SLMS LOGO (Autodesk Fusion 360 design; units mm, degrees)
Autodesk Fusion 360 part; units mm, degrees
sketch "Sketch1" plane through (0, 0, 0) normal (0, 1, 0) x (1, 0, 0)
  line L0 (0, 0) -> (135.4667, 0)
  line L1 (135.4667, 0) -> (135.4667, -135.4667)
  line L2 (135.4667, -135.4667) -> (0, -135.4667)
  line L3 (0, -135.4667) -> (0, 0)
  line L4 (27.5167, -27.5167) -> (48.6833, -27.5167)
  line L5 (48.6833, -27.5167) -> (65.8283, -56.0917)
  line L6 (65.8283, -56.0917) -> (53.1283, -77.2583)
  line L7 (53.1283, -77.2583) -> (48.6833, -69.85)
  line L8 (48.6833, -69.85) -> (48.6833, -107.95)
  line L9 (48.6833, -107.95) -> (27.5167, -107.95)
  line L10 (27.5167, -107.95) -> (27.5167, -103.7167)
  line L11 (27.5167, -103.7167) -> (31.75, -103.7167)
  line L12 (31.75, -103.7167) -> (31.75, -101.6)
  line L13 (31.75, -101.6) -> (27.5167, -101.6)
  line L14 (27.5167, -101.6) -> (27.5167, -97.3667)
  line L15 (27.5167, -97.3667) -> (35.9833, -97.3667)
  line L16 (35.9833, -97.3667) -> (35.9833, -95.25)
  line L17 (35.9833, -95.25) -> (27.5167, -95.25)
  line L18 (27.5167, -95.25) -> (27.5167, -91.0167)
  line L19 (27.5167, -91.0167) -> (31.75, -91.0167)
  line L20 (31.75, -91.0167) -> (31.75, -88.9)
  line L21 (31.75, -88.9) -> (27.5167, -88.9)
  line L22 (27.5167, -88.9) -> (27.5167, -84.6667)
  line L23 (27.5167, -84.6667) -> (31.75, -84.6667)
  line L24 (31.75, -84.6667) -> (31.75, -82.55)
  line L25 (31.75, -82.55) -> (27.5167, -82.55)
  line L26 (27.5167, -82.55) -> (27.5167, -78.3167)
  line L27 (27.5167, -78.3167) -> (35.9833, -78.3167)
  line L28 (35.9833, -78.3167) -> (35.9833, -76.2)
  line L29 (35.9833, -76.2) -> (27.5167, -76.2)
  line L30 (27.5167, -76.2) -> (27.5167, -71.9667)
  line L31 (27.5167, -71.9667) -> (31.75, -71.9667)
  line L32 (31.75, -71.9667) -> (31.75, -69.85)
  line L33 (31.75, -69.85) -> (27.5167, -69.85)
  line L34 (27.5167, -69.85) -> (27.5167, -65.6167)
  line L35 (27.5167, -65.6167) -> (31.75, -65.6167)
  line L36 (31.75, -65.6167) -> (31.75, -63.5)
  line L37 (31.75, -63.5) -> (27.5167, -63.5)
  line L38 (27.5167, -63.5) -> (27.5167, -59.2667)
  line L39 (27.5167, -59.2667) -> (35.9833, -59.2667)
  line L40 (35.9833, -59.2667) -> (35.9833, -57.15)
  line L41 (35.9833, -57.15) -> (27.5167, -57.15)
  line L42 (27.5167, -57.15) -> (27.5167, -52.9167)
  line L43 (27.5167, -52.9167) -> (31.75, -52.9167)
  line L44 (31.75, -52.9167) -> (31.75, -50.8)
  line L45 (31.75, -50.8) -> (27.5167, -50.8)
  line L46 (27.5167, -50.8) -> (27.5167, -46.5667)
  line L47 (27.5167, -46.5667) -> (31.75, -46.5667)
  line L48 (31.75, -46.5667) -> (31.75, -44.45)
  line L49 (31.75, -44.45) -> (27.5167, -44.45)
  line L50 (27.5167, -44.45) -> (27.5167, -40.2167)
  line L51 (27.5167, -40.2167) -> (35.9833, -40.2167)
  line L52 (35.9833, -40.2167) -> (35.9833, -38.1)
  line L53 (35.9833, -38.1) -> (27.5167, -38.1)
  line L54 (27.5167, -38.1) -> (27.5167, -33.8667)
  line L55 (27.5167, -33.8667) -> (31.75, -33.8667)
  line L56 (31.75, -33.8667) -> (31.75, -31.75)
  line L57 (31.75, -31.75) -> (27.5167, -31.75)
  line L58 (27.5167, -31.75) -> (27.5167, -27.5167)
  line L59 (86.7833, -27.5167) -> (55.0333, -80.4333)
  line L60 (55.0333, -80.4333) -> (67.7333, -101.6)
  line L61 (67.7333, -101.6) -> (86.7833, -69.85)
  line L62 (86.7833, -69.85) -> (86.7833, -107.95)
  line L63 (86.7833, -107.95) -> (107.95, -107.95)
  line L64 (107.95, -107.95) -> (107.95, -27.5167)
  line L65 (107.95, -27.5167) -> (86.7833, -27.5167)
  spline S0 degree 3 poles (67.7333, -82.55) (66.5692, -82.55) (65.6167, -81.5975) (65.6167, -80.4333) knots 0 0 0 0 1 1 1 1
  spline S1 degree 3 poles (65.6167, -80.4333) (65.6167, -79.2692) (66.5692, -78.3167) (67.7333, -78.3167) knots 0 0 0 0 1 1 1 1
  spline S2 degree 3 poles (67.7333, -78.3167) (68.8975, -78.3167) (69.85, -79.2692) (69.85, -80.4333) knots 0 0 0 0 1 1 1 1
  spline S3 degree 3 poles (69.85, -80.4333) (69.85, -81.5975) (68.8975, -82.55) (67.7333, -82.55) knots 0 0 0 0 1 1 1 1
  spline S4 degree 3 poles (99.4833, -97.3667) (99.4833, -98.5308) (98.5308, -99.4833) (97.3667, -99.4833) knots 0 0 0 0 1 1 1 1
  spline S5 degree 3 poles (97.3667, -99.4833) (96.2025, -99.4833) (95.25, -98.5308) (95.25, -97.3667) knots 0 0 0 0 1 1 1 1
  line L66 (95.25, -97.3667) -> (95.25, -38.1)
  spline S6 degree 3 poles (95.25, -38.1) (95.25, -36.9358) (96.2025, -35.9833) (97.3667, -35.9833) knots 0 0 0 0 1 1 1 1
  spline S7 degree 3 poles (97.3667, -35.9833) (98.5308, -35.9833) (99.4833, -36.9358) (99.4833, -38.1) knots 0 0 0 0 1 1 1 1
  line L67 (99.4833, -38.1) -> (99.4833, -97.3667)
extrude "Extrude1" add sketch "Sketch1" along normal blind 1 contours L4 L5 L6 L7 L8 L9 L10 L11 L12 L13 L14 L15 L16 L17 L18 L19 L20 L21 L22 L23 L24 L25 L26 L27 L28 L29 L30 L31 L32 L33 L34 L35 L36 L37 L38 L39 L40 L41 L42 L43 L44 L45 L46 L47 L48 L49 L50 L51 L52 L53 L54 L55 L56 L57 L58 | L59 L60 L61 L62 L63 L64 L65 makes body 1 at (50.165, 0, 41.275) makes body 2 at (80.3595, 0, 58.565)
scale "Scale1" factor 2.5 about (55.0333, 1, 80.4333) bodies 1 2
scale "Scale2" factor 0.8 about (86.7833, -1.5, 75.1417) bodies 1 2
sketch "Sketch2" plane through (0, 0.5, 0) normal (0, 1, 0) x (-1, 0, 0)
sketch "Sketch3" plane through (0, 0.5, 0) normal (0, 1, 0) x (-1, 0, 0)
  circle A0 centre (-10.5, -22.5) radius 2.5
  circle A1 centre (-36, -22.5) radius 2.5
  circle A2 centre (-138, -22.5) radius 2.5
  circle A3 centre (-163.5, -22.5) radius 2.5
  circle A4 centre (-10.5, -9.75) radius 2.5
  circle A5 centre (-36, -9.75) radius 2.5
  circle A6 centre (-138, -9.75) radius 2.5
  circle A7 centre (-163.5, -9.75) radius 2.5
  circle A8 centre (-10.5, 3) radius 2.5
  circle A9 centre (-36, 3) radius 2.5
  circle A10 centre (-61.5, 3) radius 2.5
  circle A11 centre (-112.5, 3) radius 2.5
  circle A12 centre (-138, 3) radius 2.5
  circle A13 centre (-163.5, 3) radius 2.5
  circle A14 centre (-10.5, 15.75) radius 2.5
  circle A15 centre (-36, 15.75) radius 2.5
  circle A16 centre (-61.5, 15.75) radius 2.5
  circle A17 centre (-112.5, 15.75) radius 2.5
  circle A18 centre (-138, 15.75) radius 2.5
  circle A19 centre (-163.5, 15.75) radius 2.5
  circle A20 centre (-10.5, 28.5) radius 2.5
  circle A21 centre (-36, 28.5) radius 2.5
  circle A22 centre (-61.5, 28.5) radius 2.5
  circle A23 centre (-112.5, 28.5) radius 2.5
  circle A24 centre (-138, 28.5) radius 2.5
  circle A25 centre (-163.5, 28.5) radius 2.5
  circle A26 centre (-10.5, 41.25) radius 2.5
  circle A27 centre (-36, 41.25) radius 2.5
  circle A28 centre (-61.5, 41.25) radius 2.5
  circle A29 centre (-112.5, 41.25) radius 2.5
  circle A30 centre (-138, 41.25) radius 2.5
  circle A31 centre (-163.5, 41.25) radius 2.5
  circle A32 centre (-10.5, 54) radius 2.5
  circle A33 centre (-36, 54) radius 2.5
  circle A34 centre (-61.5, 54) radius 2.5
  circle A35 centre (-87, 54) radius 2.5
  circle A36 centre (-112.5, 54) radius 2.5
  circle A37 centre (-138, 54) radius 2.5
  circle A38 centre (-163.5, 54) radius 2.5
  circle A39 centre (-10.5, 66.75) radius 2.5
  circle A40 centre (-36, 66.75) radius 2.5
  circle A41 centre (-87, 66.75) radius 2.5
  circle A42 centre (-112.5, 66.75) radius 2.5
  circle A43 centre (-138, 66.75) radius 2.5
  circle A44 centre (-163.5, 66.75) radius 2.5
  circle A45 centre (-10.5, 79.5) radius 2.5
  circle A46 centre (-36, 79.5) radius 2.5
  circle A47 centre (-138, 79.5) radius 2.5
  circle A48 centre (-163.5, 79.5) radius 2.5
  circle A49 centre (-10.5, 92.25) radius 2.5
  circle A50 centre (-36, 92.25) radius 2.5
  circle A51 centre (-87, 92.25) radius 2.5
  circle A52 centre (-138, 92.25) radius 2.5
  circle A53 centre (-163.5, 92.25) radius 2.5
  circle A54 centre (-10.5, 105) radius 2.5
  circle A55 centre (-36, 105) radius 2.5
  circle A56 centre (-87, 105) radius 2.5
  circle A57 centre (-138, 105) radius 2.5
  circle A58 centre (-163.5, 105) radius 2.5
  circle A59 centre (-10.5, 117.75) radius 2.5
  circle A60 centre (-36, 117.75) radius 2.5
  circle A61 centre (-138, 117.75) radius 2.5
  circle A62 centre (-163.5, 117.75) radius 2.5
  circle A63 centre (-10.5, 130.5) radius 2.5
  circle A64 centre (-36, 130.5) radius 2.5
  circle A65 centre (-138, 130.5) radius 2.5
  circle A66 centre (-163.5, 130.5) radius 2.5
  dimension "d11" = 5
  dimension "d14" = -153
  dimension "d15" = 153
  measures "d11" diameter of A0
sketch "Sketch8" plane through (0, 0.5, 0) normal (0, 1, 0) x (-1, 0, 0)
  line L0 (-6.35, -17.9917) -> (-14.8167, -17.9917)
  line L1 (-14.8167, -17.9917) -> (-14.8167, -13.7583)
  line L2 (-14.8167, -13.7583) -> (-6.35, -13.7583)
  line L3 (-6.35, -13.7583) -> (-6.35, -5.2917)
  line L4 (-6.35, -5.2917) -> (-23.2833, -5.2917)
  line L5 (-23.2833, -5.2917) -> (-23.2833, -1.0583)
  line L6 (-23.2833, -1.0583) -> (-6.35, -1.0583)
  line L7 (-6.35, -1.0583) -> (-6.35, 7.4083)
  line L8 (-6.35, 7.4083) -> (-14.8167, 7.4083)
  line L9 (-14.8167, 7.4083) -> (-14.8167, 11.6417)
  line L10 (-14.8167, 11.6417) -> (-6.35, 11.6417)
  line L11 (-6.35, 11.6417) -> (-6.35, 20.1083)
  line L12 (-6.35, 20.1083) -> (-14.8167, 20.1083)
  line L13 (-14.8167, 20.1083) -> (-14.8167, 24.3417)
  line L14 (-14.8167, 24.3417) -> (-6.35, 24.3417)
  line L15 (-6.35, 24.3417) -> (-6.35, 32.8083)
  line L16 (-6.35, 32.8083) -> (-23.2833, 32.8083)
  line L17 (-23.2833, 32.8083) -> (-23.2833, 37.0417)
  line L18 (-23.2833, 37.0417) -> (-6.35, 37.0417)
  line L19 (-6.35, 37.0417) -> (-6.35, 45.5083)
  line L20 (-6.35, 45.5083) -> (-14.8167, 45.5083)
  line L21 (-14.8167, 45.5083) -> (-14.8167, 49.7417)
  line L22 (-14.8167, 49.7417) -> (-6.35, 49.7417)
  line L23 (-6.35, 49.7417) -> (-6.35, 58.2083)
  line L24 (-6.35, 58.2083) -> (-14.8167, 58.2083)
  line L25 (-14.8167, 58.2083) -> (-14.8167, 62.4417)
  line L26 (-14.8167, 62.4417) -> (-6.35, 62.4417)
  line L27 (-6.35, 62.4417) -> (-6.35, 70.9083)
  line L28 (-6.35, 70.9083) -> (-23.2833, 70.9083)
  line L29 (-23.2833, 70.9083) -> (-23.2833, 75.1417)
  line L30 (-23.2833, 75.1417) -> (-6.35, 75.1417)
  line L31 (-6.35, 75.1417) -> (-6.35, 83.6083)
  line L32 (-6.35, 83.6083) -> (-14.8167, 83.6083)
  line L33 (-14.8167, 83.6083) -> (-14.8167, 87.8417)
  line L34 (-14.8167, 87.8417) -> (-6.35, 87.8417)
  line L35 (-6.35, 87.8417) -> (-6.35, 96.3083)
  line L36 (-6.35, 96.3083) -> (-14.8167, 96.3083)
  line L37 (-14.8167, 96.3083) -> (-14.8167, 100.5417)
  line L38 (-14.8167, 100.5417) -> (-6.35, 100.5417)
  line L39 (-6.35, 100.5417) -> (-6.35, 109.0083)
  line L40 (-6.35, 109.0083) -> (-23.2833, 109.0083)
  line L41 (-23.2833, 109.0083) -> (-23.2833, 113.2417)
  line L42 (-23.2833, 113.2417) -> (-6.35, 113.2417)
  line L43 (-6.35, 113.2417) -> (-6.35, 121.7083)
  line L44 (-6.35, 121.7083) -> (-14.8167, 121.7083)
  line L45 (-14.8167, 121.7083) -> (-14.8167, 125.9417)
  line L46 (-14.8167, 125.9417) -> (-6.35, 125.9417)
  line L47 (-6.35, 125.9417) -> (-6.35, 134.4083)
  line L48 (-6.35, 134.4083) -> (-48.6833, 134.4083)
  line L49 (-48.6833, 134.4083) -> (-48.6833, 58.2083)
  line L50 (-48.6833, 58.2083) -> (-57.5733, 73.025)
  line L51 (-57.5733, 73.025) -> (-82.9733, 30.6917)
  line L52 (-82.9733, 30.6917) -> (-48.6833, -26.4583)
  line L53 (-48.6833, -26.4583) -> (-6.35, -26.4583)
  line L54 (-6.35, -26.4583) -> (-6.35, -17.9917)
  line L55 (-6.35, 134.4083) -> (-167.2167, 134.4083)
  line L56 (-167.2167, 134.4083) -> (-167.2167, 144.4083)
  line L57 (-167.2167, 144.4083) -> (-6.35, 144.4083)
  line L58 (-6.35, 144.4083) -> (-6.35, 134.4083)
  dimension "d39" = 10
  constraint horizontal L55
  constraint vertical L56
  constraint horizontal L57
  constraint vertical L58
  constraint coincident L47.end L48.start
  measures "d39" distance of L47.end L57.end
extrude "Extrude9" add sketch "Sketch8" against normal blind 40 separate body contours L48 L55 L56 L57 L58 makes body 3
sketch "Sketch4" plane through (0, 0.5, 0) normal (0, 1, 0) x (-1, 0, 0)
  circle A0 centre (-23, -10) radius 1.5
  circle A1 centre (-48.5, -10) radius 1.5
  circle A2 centre (-125, -10) radius 1.5
  circle A3 centre (-150.5, -10) radius 1.5
  circle A4 centre (-23, 15.5) radius 1.5
  circle A5 centre (-48.5, 15.5) radius 1.5
  circle A6 centre (-125, 15.5) radius 1.5
  circle A7 centre (-23, 41) radius 1.5
  circle A8 centre (-48.5, 41) radius 1.5
  circle A9 centre (-74, 41) radius 1.5
  circle A10 centre (-99.5, 41) radius 1.5
  circle A11 centre (-125, 41) radius 1.5
  circle A12 centre (-23, 66.5) radius 1.5
  circle A13 centre (-74, 66.5) radius 1.5
  circle A14 centre (-99.5, 66.5) radius 1.5
  circle A15 centre (-23, 92) radius 1.5
  circle A16 centre (-74, 92) radius 1.5
  circle A17 centre (-99.5, 92) radius 1.5
  circle A18 centre (-23, 117.5) radius 1.5
  circle A19 centre (-150.5, 117.5) radius 1.5
  point P0 (-10.5, -22.5)
  dimension "d17" = 3
  dimension "d20" = -153
  dimension "d21" = 153
  measures "d17" diameter of A0
extrude "Extrude4" [suppressed]
shell "Shell2" [suppressed]
extrude "Extrude5" [suppressed]
extrude "Extrude6" [suppressed]
sketch "Sketch7" plane through (0, -1.5, 0) normal (0, -1, 0) x (1, 0, 0)
  arc A0 (12.809, 118.7083) -> (12.4937, 116.2417) centre (10.5, 117.75) ccw
  line L0 (12.809, 118.7083) -> (17.8167, 118.7083)
  line L1 (17.8167, 118.7083) -> (17.8167, 128.9417)
  line L2 (17.8167, 128.9417) -> (12.4549, 128.9417)
  arc A1 (12.8291, 131.4083) -> (12.4549, 128.9417) centre (10.5, 130.5) ccw
  line L3 (12.8291, 131.4083) -> (33.6709, 131.4083)
  arc A2 (38.3291, 131.4083) -> (33.6709, 131.4083) centre (36, 130.5) ccw
  line L4 (38.3291, 131.4083) -> (45.6833, 131.4083)
  line L5 (45.6833, 131.4083) -> (45.6833, 47.3774)
  line L6 (45.6833, 47.3774) -> (57.5733, 67.194)
  line L7 (57.5733, 67.194) -> (72.7725, 41.8621)
  arc A3 (74.183, 39.5112) -> (72.7725, 41.8621) centre (74, 41) ccw
  line L8 (74.183, 39.5112) -> (79.4748, 30.6917)
  line L9 (79.4748, 30.6917) -> (63.6376, 4.2964)
  arc A4 (61.362, 0.5038) -> (63.6376, 4.2964) centre (61.5, 3) ccw
  line L10 (61.362, 0.5038) -> (46.9848, -23.4583)
  line L11 (46.9848, -23.4583) -> (38.309, -23.4583)
  arc A5 (33.691, -23.4583) -> (38.309, -23.4583) centre (36, -22.5) ccw
  line L12 (33.691, -23.4583) -> (12.809, -23.4583)
  arc A6 (12.4937, -20.9917) -> (12.809, -23.4583) centre (10.5, -22.5) ccw
  line L13 (12.4937, -20.9917) -> (17.8167, -20.9917)
  line L14 (17.8167, -20.9917) -> (17.8167, -10.7583)
  line L15 (17.8167, -10.7583) -> (12.7876, -10.7583)
  arc A7 (12.5306, -8.2917) -> (12.7876, -10.7583) centre (10.5, -9.75) ccw
  line L16 (12.5306, -8.2917) -> (26.2833, -8.2917)
  line L17 (26.2833, -8.2917) -> (26.2833, 1.9417)
  line L18 (26.2833, 1.9417) -> (12.7649, 1.9417)
  arc A8 (12.5656, 4.4083) -> (12.7649, 1.9417) centre (10.5, 3) ccw
  line L19 (12.5656, 4.4083) -> (17.8167, 4.4083)
  line L20 (17.8167, 4.4083) -> (17.8167, 14.6417)
  line L21 (17.8167, 14.6417) -> (12.7409, 14.6417)
  arc A9 (12.5988, 17.1083) -> (12.7409, 14.6417) centre (10.5, 15.75) ccw
  line L22 (12.5988, 17.1083) -> (17.8167, 17.1083)
  line L23 (17.8167, 17.1083) -> (17.8167, 27.3417)
  line L24 (17.8167, 27.3417) -> (12.7155, 27.3417)
  arc A10 (12.6303, 29.8083) -> (12.7155, 27.3417) centre (10.5, 28.5) ccw
  line L25 (12.6303, 29.8083) -> (26.2833, 29.8083)
  line L26 (26.2833, 29.8083) -> (26.2833, 40.0417)
  line L27 (26.2833, 40.0417) -> (24.1539, 40.0417)
  arc A11 (21.8461, 40.0417) -> (24.1539, 40.0417) centre (23, 41) ccw
  line L28 (21.8461, 40.0417) -> (12.6886, 40.0417)
  arc A12 (12.6602, 42.5083) -> (12.6886, 40.0417) centre (10.5, 41.25) ccw
  line L29 (12.6602, 42.5083) -> (17.8167, 42.5083)
  line L30 (17.8167, 42.5083) -> (17.8167, 52.7417)
  line L31 (17.8167, 52.7417) -> (12.6602, 52.7417)
  arc A13 (12.6886, 55.2083) -> (12.6602, 52.7417) centre (10.5, 54) ccw
  line L32 (12.6886, 55.2083) -> (17.8167, 55.2083)
  line L33 (17.8167, 55.2083) -> (17.8167, 65.4417)
  line L34 (17.8167, 65.4417) -> (12.6303, 65.4417)
  arc A14 (12.7155, 67.9083) -> (12.6303, 65.4417) centre (10.5, 66.75) ccw
  line L35 (12.7155, 67.9083) -> (22.4837, 67.9083)
  arc A15 (23.5163, 67.9083) -> (22.4837, 67.9083) centre (23, 66.5) ccw
  line L36 (23.5163, 67.9083) -> (26.2833, 67.9083)
  line L37 (26.2833, 67.9083) -> (26.2833, 78.1417)
  line L38 (26.2833, 78.1417) -> (12.5988, 78.1417)
  arc A16 (12.7409, 80.6083) -> (12.5988, 78.1417) centre (10.5, 79.5) ccw
  line L39 (12.7409, 80.6083) -> (17.8167, 80.6083)
  line L40 (17.8167, 80.6083) -> (17.8167, 90.8417)
  line L41 (17.8167, 90.8417) -> (12.5656, 90.8417)
  arc A17 (12.7649, 93.3083) -> (12.5656, 90.8417) centre (10.5, 92.25) ccw
  line L42 (12.7649, 93.3083) -> (17.8167, 93.3083)
  line L43 (17.8167, 93.3083) -> (17.8167, 103.5417)
  line L44 (17.8167, 103.5417) -> (12.5306, 103.5417)
  arc A18 (12.7876, 106.0083) -> (12.5306, 103.5417) centre (10.5, 105) ccw
  line L45 (12.7876, 106.0083) -> (26.2833, 106.0083)
  line L46 (26.2833, 106.0083) -> (26.2833, 116.2417)
  line L47 (26.2833, 116.2417) -> (23.8165, 116.2417)
  arc A19 (22.1835, 116.2417) -> (23.8165, 116.2417) centre (23, 117.5) ccw
  line L48 (22.1835, 116.2417) -> (12.4937, 116.2417)
  line L49 (14.8167, -17.9917) -> (6.35, -17.9917)
  line L50 (6.35, -17.9917) -> (6.35, -26.4583)
  line L51 (6.35, -26.4583) -> (48.6833, -26.4583)
  line L52 (48.6833, -26.4583) -> (82.9733, 30.6917)
  line L53 (82.9733, 30.6917) -> (57.5733, 73.025)
  line L54 (57.5733, 73.025) -> (48.6833, 58.2083)
  line L55 (48.6833, 58.2083) -> (48.6833, 134.4083)
  line L56 (48.6833, 134.4083) -> (6.35, 134.4083)
  line L57 (6.35, 134.4083) -> (6.35, 125.9417)
  line L58 (6.35, 125.9417) -> (14.8167, 125.9417)
  line L59 (14.8167, 125.9417) -> (14.8167, 121.7083)
  line L60 (14.8167, 121.7083) -> (6.35, 121.7083)
  line L61 (6.35, 121.7083) -> (6.35, 113.2417)
  line L62 (6.35, 113.2417) -> (23.2833, 113.2417)
  line L63 (23.2833, 113.2417) -> (23.2833, 109.0083)
  line L64 (23.2833, 109.0083) -> (6.35, 109.0083)
  line L65 (6.35, 109.0083) -> (6.35, 100.5417)
  line L66 (6.35, 100.5417) -> (14.8167, 100.5417)
  line L67 (14.8167, 100.5417) -> (14.8167, 96.3083)
  line L68 (14.8167, 96.3083) -> (6.35, 96.3083)
  line L69 (6.35, 96.3083) -> (6.35, 87.8417)
  line L70 (6.35, 87.8417) -> (14.8167, 87.8417)
  line L71 (14.8167, 87.8417) -> (14.8167, 83.6083)
  line L72 (14.8167, 83.6083) -> (6.35, 83.6083)
  line L73 (6.35, 83.6083) -> (6.35, 75.1417)
  line L74 (6.35, 75.1417) -> (23.2833, 75.1417)
  line L75 (23.2833, 75.1417) -> (23.2833, 70.9083)
  line L76 (23.2833, 70.9083) -> (6.35, 70.9083)
  line L77 (6.35, 70.9083) -> (6.35, 62.4417)
  line L78 (6.35, 62.4417) -> (14.8167, 62.4417)
  line L79 (14.8167, 62.4417) -> (14.8167, 58.2083)
  line L80 (14.8167, 58.2083) -> (6.35, 58.2083)
  line L81 (6.35, 58.2083) -> (6.35, 49.7417)
  line L82 (6.35, 49.7417) -> (14.8167, 49.7417)
  line L83 (14.8167, 49.7417) -> (14.8167, 45.5083)
  line L84 (14.8167, 45.5083) -> (6.35, 45.5083)
  line L85 (6.35, 45.5083) -> (6.35, 37.0417)
  line L86 (6.35, 37.0417) -> (23.2833, 37.0417)
  line L87 (23.2833, 37.0417) -> (23.2833, 32.8083)
  line L88 (23.2833, 32.8083) -> (6.35, 32.8083)
  line L89 (6.35, 32.8083) -> (6.35, 24.3417)
  line L90 (6.35, 24.3417) -> (14.8167, 24.3417)
  line L91 (14.8167, 24.3417) -> (14.8167, 20.1083)
  line L92 (14.8167, 20.1083) -> (6.35, 20.1083)
  line L93 (6.35, 20.1083) -> (6.35, 11.6417)
  line L94 (6.35, 11.6417) -> (14.8167, 11.6417)
  line L95 (14.8167, 11.6417) -> (14.8167, 7.4083)
  line L96 (14.8167, 7.4083) -> (6.35, 7.4083)
  line L97 (6.35, 7.4083) -> (6.35, -1.0583)
  line L98 (6.35, -1.0583) -> (23.2833, -1.0583)
  line L99 (23.2833, -1.0583) -> (23.2833, -5.2917)
  line L100 (23.2833, -5.2917) -> (6.35, -5.2917)
  line L101 (6.35, -5.2917) -> (6.35, -13.7583)
  line L102 (6.35, -13.7583) -> (14.8167, -13.7583)
  line L103 (14.8167, -13.7583) -> (14.8167, -17.9917)
  line L104 (124.8833, -26.4583) -> (61.3833, 79.375)
  line L105 (82.9733, 30.6917) -> (90.5933, 30.6917)
  line L106 (81.791, 32.6623) -> (89.411, 32.6623)
  line L107 (89.411, 32.6623) -> (90.5933, 30.6917)
  line L108 (82.9733, 30.6917) -> (81.791, 32.6623)
  constraint coincident L52.end L53.start
  constraint coincident L104 L105.end
  constraint horizontal L105
  constraint coincident L53 L106.start
  constraint coincident L104 L106.end
  constraint parallel L105 L106
extrude "Extrude7" [suppressed]
extrude "Extrude8" [suppressed]
sketch "Sketch6" plane through (0, -1.5, 0) normal (0, -1, 0) x (1, 0, 0)
  arc A0 (12.809, 118.7083) -> (12.4937, 116.2417) centre (10.5, 117.75) ccw
  line L0 (12.809, 118.7083) -> (17.8167, 118.7083)
  line L1 (17.8167, 118.7083) -> (17.8167, 128.9417)
  line L2 (17.8167, 128.9417) -> (12.4549, 128.9417)
  arc A1 (12.8291, 131.4083) -> (12.4549, 128.9417) centre (10.5, 130.5) ccw
  line L3 (12.8291, 131.4083) -> (33.6709, 131.4083)
  arc A2 (38.3291, 131.4083) -> (33.6709, 131.4083) centre (36, 130.5) ccw
  line L4 (38.3291, 131.4083) -> (45.6833, 131.4083)
  line L5 (45.6833, 131.4083) -> (45.6833, 47.3774)
  line L6 (45.6833, 47.3774) -> (57.5733, 67.194)
  line L7 (57.5733, 67.194) -> (72.7725, 41.8621)
  arc A3 (74.183, 39.5112) -> (72.7725, 41.8621) centre (74, 41) ccw
  line L8 (74.183, 39.5112) -> (79.4748, 30.6917)
  line L9 (79.4748, 30.6917) -> (63.6376, 4.2964)
  arc A4 (61.362, 0.5038) -> (63.6376, 4.2964) centre (61.5, 3) ccw
  line L10 (61.362, 0.5038) -> (46.9848, -23.4583)
  line L11 (46.9848, -23.4583) -> (38.309, -23.4583)
  arc A5 (33.691, -23.4583) -> (38.309, -23.4583) centre (36, -22.5) ccw
  line L12 (33.691, -23.4583) -> (12.809, -23.4583)
  arc A6 (12.4937, -20.9917) -> (12.809, -23.4583) centre (10.5, -22.5) ccw
  line L13 (12.4937, -20.9917) -> (17.8167, -20.9917)
  line L14 (17.8167, -20.9917) -> (17.8167, -10.7583)
  line L15 (17.8167, -10.7583) -> (12.7876, -10.7583)
  arc A7 (12.5306, -8.2917) -> (12.7876, -10.7583) centre (10.5, -9.75) ccw
  line L16 (12.5306, -8.2917) -> (26.2833, -8.2917)
  line L17 (26.2833, -8.2917) -> (26.2833, 1.9417)
  line L18 (26.2833, 1.9417) -> (12.7649, 1.9417)
  arc A8 (12.5656, 4.4083) -> (12.7649, 1.9417) centre (10.5, 3) ccw
  line L19 (12.5656, 4.4083) -> (17.8167, 4.4083)
  line L20 (17.8167, 4.4083) -> (17.8167, 14.6417)
  line L21 (17.8167, 14.6417) -> (12.7409, 14.6417)
  arc A9 (12.5988, 17.1083) -> (12.7409, 14.6417) centre (10.5, 15.75) ccw
  line L22 (12.5988, 17.1083) -> (17.8167, 17.1083)
  line L23 (17.8167, 17.1083) -> (17.8167, 27.3417)
  line L24 (17.8167, 27.3417) -> (12.7155, 27.3417)
  arc A10 (12.6303, 29.8083) -> (12.7155, 27.3417) centre (10.5, 28.5) ccw
  line L25 (12.6303, 29.8083) -> (26.2833, 29.8083)
  line L26 (26.2833, 29.8083) -> (26.2833, 40.0417)
  line L27 (26.2833, 40.0417) -> (24.1539, 40.0417)
  arc A11 (21.8461, 40.0417) -> (24.1539, 40.0417) centre (23, 41) ccw
  line L28 (21.8461, 40.0417) -> (12.6886, 40.0417)
  arc A12 (12.6602, 42.5083) -> (12.6886, 40.0417) centre (10.5, 41.25) ccw
  line L29 (12.6602, 42.5083) -> (17.8167, 42.5083)
  line L30 (17.8167, 42.5083) -> (17.8167, 52.7417)
  line L31 (17.8167, 52.7417) -> (12.6602, 52.7417)
  arc A13 (12.6886, 55.2083) -> (12.6602, 52.7417) centre (10.5, 54) ccw
  line L32 (12.6886, 55.2083) -> (17.8167, 55.2083)
  line L33 (17.8167, 55.2083) -> (17.8167, 65.4417)
  line L34 (17.8167, 65.4417) -> (12.6303, 65.4417)
  arc A14 (12.7155, 67.9083) -> (12.6303, 65.4417) centre (10.5, 66.75) ccw
  line L35 (12.7155, 67.9083) -> (22.4837, 67.9083)
  arc A15 (23.5163, 67.9083) -> (22.4837, 67.9083) centre (23, 66.5) ccw
  line L36 (23.5163, 67.9083) -> (26.2833, 67.9083)
  line L37 (26.2833, 67.9083) -> (26.2833, 78.1417)
  line L38 (26.2833, 78.1417) -> (12.5988, 78.1417)
  arc A16 (12.7409, 80.6083) -> (12.5988, 78.1417) centre (10.5, 79.5) ccw
  line L39 (12.7409, 80.6083) -> (17.8167, 80.6083)
  line L40 (17.8167, 80.6083) -> (17.8167, 90.8417)
  line L41 (17.8167, 90.8417) -> (12.5656, 90.8417)
  arc A17 (12.7649, 93.3083) -> (12.5656, 90.8417) centre (10.5, 92.25) ccw
  line L42 (12.7649, 93.3083) -> (17.8167, 93.3083)
  line L43 (17.8167, 93.3083) -> (17.8167, 103.5417)
  line L44 (17.8167, 103.5417) -> (12.5306, 103.5417)
  arc A18 (12.7876, 106.0083) -> (12.5306, 103.5417) centre (10.5, 105) ccw
  line L45 (12.7876, 106.0083) -> (26.2833, 106.0083)
  line L46 (26.2833, 106.0083) -> (26.2833, 116.2417)
  line L47 (26.2833, 116.2417) -> (23.8165, 116.2417)
  arc A19 (22.1835, 116.2417) -> (23.8165, 116.2417) centre (23, 117.5) ccw
  line L48 (22.1835, 116.2417) -> (12.4937, 116.2417)
  line L49 (14.8167, -17.9917) -> (6.35, -17.9917)
  line L50 (6.35, -17.9917) -> (6.35, -26.4583)
  line L51 (6.35, -26.4583) -> (48.6833, -26.4583)
  line L52 (48.6833, -26.4583) -> (82.9733, 30.6917)
  line L53 (82.9733, 30.6917) -> (57.5733, 73.025)
  line L54 (57.5733, 73.025) -> (48.6833, 58.2083)
  line L55 (48.6833, 58.2083) -> (48.6833, 134.4083)
  line L56 (48.6833, 134.4083) -> (6.35, 134.4083)
  line L57 (6.35, 134.4083) -> (6.35, 125.9417)
  line L58 (6.35, 125.9417) -> (14.8167, 125.9417)
  line L59 (14.8167, 125.9417) -> (14.8167, 121.7083)
  line L60 (14.8167, 121.7083) -> (6.35, 121.7083)
  line L61 (6.35, 121.7083) -> (6.35, 113.2417)
  line L62 (6.35, 113.2417) -> (23.2833, 113.2417)
  line L63 (23.2833, 113.2417) -> (23.2833, 109.0083)
  line L64 (23.2833, 109.0083) -> (6.35, 109.0083)
  line L65 (6.35, 109.0083) -> (6.35, 100.5417)
  line L66 (6.35, 100.5417) -> (14.8167, 100.5417)
  line L67 (14.8167, 100.5417) -> (14.8167, 96.3083)
  line L68 (14.8167, 96.3083) -> (6.35, 96.3083)
  line L69 (6.35, 96.3083) -> (6.35, 87.8417)
  line L70 (6.35, 87.8417) -> (14.8167, 87.8417)
  line L71 (14.8167, 87.8417) -> (14.8167, 83.6083)
  line L72 (14.8167, 83.6083) -> (6.35, 83.6083)
  line L73 (6.35, 83.6083) -> (6.35, 75.1417)
  line L74 (6.35, 75.1417) -> (23.2833, 75.1417)
  line L75 (23.2833, 75.1417) -> (23.2833, 70.9083)
  line L76 (23.2833, 70.9083) -> (6.35, 70.9083)
  line L77 (6.35, 70.9083) -> (6.35, 62.4417)
  line L78 (6.35, 62.4417) -> (14.8167, 62.4417)
  line L79 (14.8167, 62.4417) -> (14.8167, 58.2083)
  line L80 (14.8167, 58.2083) -> (6.35, 58.2083)
  line L81 (6.35, 58.2083) -> (6.35, 49.7417)
  line L82 (6.35, 49.7417) -> (14.8167, 49.7417)
  line L83 (14.8167, 49.7417) -> (14.8167, 45.5083)
  line L84 (14.8167, 45.5083) -> (6.35, 45.5083)
  line L85 (6.35, 45.5083) -> (6.35, 37.0417)
  line L86 (6.35, 37.0417) -> (23.2833, 37.0417)
  line L87 (23.2833, 37.0417) -> (23.2833, 32.8083)
  line L88 (23.2833, 32.8083) -> (6.35, 32.8083)
  line L89 (6.35, 32.8083) -> (6.35, 24.3417)
  line L90 (6.35, 24.3417) -> (14.8167, 24.3417)
  line L91 (14.8167, 24.3417) -> (14.8167, 20.1083)
  line L92 (14.8167, 20.1083) -> (6.35, 20.1083)
  line L93 (6.35, 20.1083) -> (6.35, 11.6417)
  line L94 (6.35, 11.6417) -> (14.8167, 11.6417)
  line L95 (14.8167, 11.6417) -> (14.8167, 7.4083)
  line L96 (14.8167, 7.4083) -> (6.35, 7.4083)
  line L97 (6.35, 7.4083) -> (6.35, -1.0583)
  line L98 (6.35, -1.0583) -> (23.2833, -1.0583)
  line L99 (23.2833, -1.0583) -> (23.2833, -5.2917)
  line L100 (23.2833, -5.2917) -> (6.35, -5.2917)
  line L101 (6.35, -5.2917) -> (6.35, -13.7583)
  line L102 (6.35, -13.7583) -> (14.8167, -13.7583)
  line L103 (14.8167, -13.7583) -> (14.8167, -17.9917)
  line L104 (8.0283, 132.9322) -> (38.5, 132.9322)
  line L105 (38.5, 132.9322) -> (38.5, -25)
  line L106 (38.5, -25) -> (8.0283, -25)
  line L107 (8.0283, -25) -> (8.0283, 132.9322)
  line L108 (71.8895, 43.3338) -> (74.8225, 43.3338)
  line L109 (74.8225, 43.3338) -> (74.8225, 38.4454)
  line L110 (74.8225, 38.4454) -> (71.8895, 38.4454)
  line L111 (71.8895, 38.4454) -> (71.8895, 43.3338)
  line L112 (57, 6) -> (63.6437, 6)
  line L113 (63.6437, 6) -> (63.6437, 0.5038)
  line L114 (63.6437, 0.5038) -> (57, 0.5038)
  line L115 (57, 0.5038) -> (57, 6)
  constraint horizontal L104
  constraint vertical L105
  constraint horizontal L106
  constraint vertical L107
  constraint horizontal L108
  constraint vertical L109
  constraint horizontal L110
  constraint vertical L111
  constraint coincident L8 L109.end
  constraint coincident L7 L108.start
  constraint horizontal L112
  constraint vertical L113
  constraint horizontal L114
  constraint vertical L115
